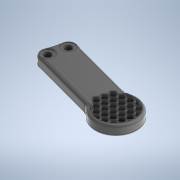
# Autodesk Inventor part: RearBumper
Saved by Autodesk Inventor 2020 (Build 240168000, 168)
## iProperties
Part Number: RearBumper
Material: PC/ABS プラスチック
Document SubType Name: Modeling
Designer: Masato Kubotera
Density: 0.357273 g/cm^3
Appearance: 滑らか - 黒
Description: TPU
Author: Masato Kubotera
Autodesk Inventor part; units mm, degrees
ref_plane "YZ Plane" through (0, 0, 0) normal (1, 0, 0) x (0, 1, 0)
ref_plane "XZ Plane" through (0, 0, 0) normal (0, 1, 0) x (-1, 0, 0)
ref_plane "XY Plane" through (0, 0, 0) normal (0, 0, 1) x (1, 0, 0)
derived "Trunk_basis.ipt"
sketch "スケッチ1" plane through (0, 0, 0) normal (0, 1, 0) x (-1, 0, 0)
  line L0 (0, 22) -> (0, -142.9) construction
  circle A0 centre (5, 0) radius 10.5 construction
  line L1 (-7, 16) -> (36, 16) construction
  line L2 (36, 16) -> (36, -16) construction
  line L3 (36, -16) -> (-7, -16) construction
  line L4 (-7, -16) -> (-7, 16) construction
  line L5 (-7, 16) -> (36, -16) construction
  line L6 (36, 16) -> (-7, -16) construction
  line L7 (33, 13.5) -> (6, 13.5) construction
  line L8 (6, 13.5) -> (6, -13.5) construction
  line L9 (6, -13.5) -> (33, -13.5) construction
  line L10 (33, -13.5) -> (33, 13.5) construction
  line L11 (33, 13.5) -> (6, -13.5) construction
  line L12 (6, 13.5) -> (33, -13.5) construction
  line L13 (-7, 0) -> (36, 0) construction
  arc A1 (5, 16) -> (-7, 10.583) centre (5, 0) ccw construction
  line L14 (43.75, -16.25) -> (5, -16.25)
  line L15 (5, 16.25) -> (43.75, 16.25)
  line L16 (44.75, 15.25) -> (44.75, -15.25)
  arc A2 (5, 16.25) -> (-6.7376, 11.2379) centre (5, 0) ccw
  arc A3 (-6.7376, 11.2379) -> (-7.25, 9.9174) centre (-6.2711, 10.2972) ccw
  circle A4 centre (6, 13.5) radius 1.35
  line L17 (19.5, 13.5) -> (19.5, -13.5) construction
  circle A5 centre (33, 13.5) radius 1.35
  line L18 (-15, 22) -> (-20, 17)
  line L19 (-20, 17) -> (-20, -19)
  line L20 (-20, -19) -> (-28.5, -27.5)
  line L21 (-28.5, -27.5) -> (-28.5, -103)
  line L22 (57.5, -22.5) -> (57.5, 17)
  line L23 (57.5, 17) -> (52.5, 22)
  line L24 (52.5, 22) -> (-15, 22)
  line L25 (-35.5597, -116.5529) -> (-28.5, -142.9)
  line L26 (-16, -139) -> (-16, -94) construction
  line L27 (-7.5, -140.4849) -> (-7.5, -142.9)
  line L28 (-7.5, -142.9) -> (7.5, -142.9)
  line L29 (7.5, -140.4849) -> (7.5, -142.9)
  arc A6 (-7.5, -140.4849) -> (-8.9849, -139) centre (-8.2425, -139.7425) ccw
  line L30 (-17.5, -138.9955) -> (-17.5, -133) construction
  line L31 (-19, -133) -> (-16, -133) construction
  line L32 (-19, -133) -> (-19, -139) construction
  line L33 (-16, -133) -> (-16, -139) construction
  line L34 (-15, 22) -> (-10, 22) construction
  line L35 (-10, 22) -> (-10, -22) construction
  line L36 (-10, -22) -> (-15, -22) construction
  line L37 (-15, -22) -> (-15, 22) construction
  line L38 (-15, 22) -> (-10, -22) construction
  line L39 (-10, 22) -> (-15, -22) construction
  line L40 (-12.5, 22) -> (-12.5, -22) construction
  line L41 (-10, 0) -> (-15, 0) construction
  circle A7 centre (-12.5, 17.75) radius 1.6
  line L42 (-15, 10) -> (-12.5, 10) construction
  line L43 (-12.5, 10) -> (-12.5, -10) construction
  line L44 (-12.5, -10) -> (-15, -10) construction
  line L45 (-15, -10) -> (-15, 10) construction
  line L46 (-15, 10) -> (-12.5, -10) construction
  line L47 (-12.5, 10) -> (-15, -10) construction
  line L48 (-12.25, 10.25) -> (-15.25, 10.25)
  line L49 (-15.25, 8.15) -> (-15.25, -8.15)
  line L50 (-15.25, -10.25) -> (-12.25, -10.25)
  line L51 (-12.25, -8.15) -> (-12.25, 8.15)
  line L52 (-12.25, 10.25) -> (-15.25, -10.25) construction
  line L53 (-15.25, 10.25) -> (-12.25, -10.25) construction
  arc A8 (-15.25, 10.25) -> (-15.25, 8.15) centre (-15.25, 9.2) ccw
  line L54 (-13.75, 10) -> (-13.75, -10) construction
  arc A9 (-12.25, 8.15) -> (-12.25, 10.25) centre (-12.25, 9.2) ccw
  circle A10 centre (-12.5, -17.75) radius 1.6
  arc A11 (-15.25, -8.15) -> (-15.25, -10.25) centre (-15.25, -9.2) ccw
  arc A12 (-12.25, -10.25) -> (-12.25, -8.15) centre (-12.25, -9.2) ccw
  line L55 (36, 14.4) -> (44.5, 14.4) construction
  line L56 (44.5, 14.4) -> (44.5, -14.4) construction
  line L57 (36, -14.4) -> (44.5, -14.4) construction
  line L58 (49.95, 7.95) -> (49.95, -7.95)
  line L59 (52.5, 0) -> (47.5, 0) construction
  line L60 (47.5, 22) -> (52.5, 22) construction
  line L61 (52.55, -7.95) -> (52.55, 7.95)
  line L62 (51.25, 10) -> (51.25, -10) construction
  line L63 (52.5, 10) -> (50, -10) construction
  line L64 (52.5, -10) -> (50, -10) construction
  line L65 (52.5, 10) -> (52.5, -10) construction
  line L66 (50, 10) -> (52.5, -10) construction
  line L67 (49.95, -10.05) -> (52.55, -10.05)
  line L68 (49.95, 10.05) -> (52.55, -10.05) construction
  line L69 (52.55, 10.05) -> (49.95, -10.05) construction
  line L70 (52.5, -22) -> (47.5, -22) construction
  line L71 (47.5, 22) -> (52.5, -22) construction
  line L72 (52.5, 22) -> (52.5, -22) construction
  line L73 (52.5, 22) -> (47.5, -22) construction
  line L74 (50, 22) -> (50, -22) construction
  line L75 (47.5, -22) -> (47.5, 22) construction
  circle A13 centre (50, -17.75) radius 1.6
  arc A14 (52.55, -10.05) -> (52.55, -7.95) centre (52.55, -9) ccw
  line L76 (50, -10) -> (50, 10) construction
  arc A15 (49.95, -7.95) -> (49.95, -10.05) centre (49.95, -9) ccw
  arc A16 (49.95, 10.05) -> (49.95, 7.95) centre (49.95, 9) ccw
  arc A17 (52.55, 7.95) -> (52.55, 10.05) centre (52.55, 9) ccw
  line L77 (50, 10) -> (52.5, 10) construction
  line L78 (52.55, 10.05) -> (49.95, 10.05)
  circle A18 centre (50, 17.75) radius 1.6
  circle A19 centre (5, 0) radius 16 construction
  arc A20 (-6.7376, -11.2379) -> (5, -16.25) centre (5, 0) ccw
  arc A21 (-7.25, -9.9174) -> (-6.7376, -11.2379) centre (-6.2711, -10.2972) ccw
  line L79 (-7.25, -9.9174) -> (-7.25, 9.9174)
  line L80 (17.5, -138.9955) -> (17.5, -133) construction
  line L81 (19, -133) -> (19, -139) construction
  line L82 (16, -133) -> (16, -139) construction
  line L83 (19, -133) -> (16, -133) construction
  circle A22 centre (6, -13.5) radius 1.35
  circle A23 centre (33, -13.5) radius 1.35
  line L84 (-25.5, -142.9) -> (-7.5, -142.9) construction
  line L85 (25.5, -142.9) -> (7.5, -142.9) construction
  line L86 (-23.5, -22.5) -> (57.5, -22.5) construction
  line L87 (57.5, -22.5) -> (57.5, -103)
  circle A24 centre (-13.5, -55) radius 1.75
  line L88 (-16.5, -59) -> (45.5, -59)
  line L89 (47.5, -61) -> (47.5, -82.5)
  line L90 (45.5, -84.5) -> (-16.5, -84.5)
  line L91 (-18.5, -82.5) -> (-18.5, -61)
  line L92 (-18.5, -59) -> (47.5, -84.5) construction
  line L93 (47.5, -59) -> (-18.5, -84.5) construction
  line L94 (-16.5, -27.5) -> (45.5, -27.5)
  line L95 (47.5, -29.5) -> (47.5, -49)
  line L96 (45.5, -51) -> (-16.5, -51)
  line L97 (-18.5, -49) -> (-18.5, -29.5)
  line L98 (-18.5, -27.5) -> (47.5, -51) construction
  line L99 (47.5, -27.5) -> (-18.5, -51) construction
  line L100 (-23.5, -108) -> (-28.5, -103)
  circle A25 centre (-20.5415, -102) radius 1.6
  line L101 (-25.7227, -96) -> (25.7227, -96)
  line L102 (25.7227, -96) -> (34.9603, -112)
  line L103 (35.5597, -116.5529) -> (28.5, -142.9)
  line L104 (-25.7227, -96) -> (-34.9603, -112)
  line L105 (57.5, -103) -> (52.5, -108)
  arc A26 (-16.5, -27.5) -> (-18.5, -29.5) centre (-16.5, -29.5) ccw
  arc A27 (-18.5, -49) -> (-16.5, -51) centre (-16.5, -49) ccw
  arc A28 (45.5, -51) -> (47.5, -49) centre (45.5, -49) ccw
  arc A29 (47.5, -29.5) -> (45.5, -27.5) centre (45.5, -29.5) ccw
  arc A30 (-16.5, -59) -> (-18.5, -61) centre (-16.5, -61) ccw
  arc A31 (-18.5, -82.5) -> (-16.5, -84.5) centre (-16.5, -82.5) ccw
  arc A32 (45.5, -84.5) -> (47.5, -82.5) centre (45.5, -82.5) ccw
  arc A33 (47.5, -61) -> (45.5, -59) centre (45.5, -61) ccw
  line L106 (-23.5, -108) -> (52.5, -108)
  line L107 (-25.5, -139) -> (-25.5, -142.9)
  line L108 (-25.5, -142.9) -> (-28.5, -142.9)
  line L109 (-17.9813, -99.3843) -> (-16.9961, -101.0907)
  line L110 (-16.9961, -102.9093) -> (-17.9813, -104.6157)
  line L111 (-19.5563, -105.525) -> (-21.5266, -105.525)
  line L112 (-23.1016, -104.6157) -> (-24.0868, -102.9093)
  line L113 (-24.0868, -101.0907) -> (-23.1016, -99.3843)
  line L114 (-21.5266, -98.475) -> (-19.5563, -98.475)
  line L115 (-16, -94) -> (16, -94) construction
  arc A34 (-24.0868, -101.0907) -> (-24.0868, -102.9093) centre (-23.5618, -102) ccw
  arc A35 (-23.1016, -104.6157) -> (-21.5266, -105.525) centre (-22.0516, -104.6157) ccw
  arc A36 (-19.5563, -105.525) -> (-17.9813, -104.6157) centre (-19.0313, -104.6157) ccw
  arc A37 (-16.9961, -102.9093) -> (-16.9961, -101.0907) centre (-17.5211, -102) ccw
  arc A38 (-17.9813, -99.3843) -> (-19.5563, -98.475) centre (-19.0313, -99.3843) ccw
  arc A39 (-21.5266, -98.475) -> (-23.1016, -99.3843) centre (-22.0516, -99.3843) ccw
  line L116 (16, -139) -> (16, -94) construction
  line L117 (16, -94) -> (-16, -94) construction
  line L118 (-25.5, -139) -> (-8.9849, -139)
  line L119 (25.5, -142.9) -> (28.5, -142.9)
  arc A40 (8.9849, -139) -> (7.5, -140.4849) centre (8.2425, -139.7425) ccw
  circle A41 centre (29.7641, -115) radius 1.25
  line L120 (33.4891, -124.2803) -> (21.898, -121.1745) construction
  line L121 (29.7641, -115) -> (25.623, -130.4548) construction
  circle A42 centre (29.7641, -115) radius 6 construction
  circle A43 centre (-20.5415, -102) radius 6 construction
  line L122 (1.9319, -109.4824) -> (7.5588, -130.4824)
  line L123 (5.6269, -133) -> (-5.6269, -133)
  line L124 (5.3151, -110.5176) -> (10.942, -131.5176)
  line L125 (12.8739, -133) -> (17.1947, -133)
  line L126 (19.1266, -131.5176) -> (24.7535, -110.5176)
  line L127 (22.8217, -108) -> (7.2469, -108)
  circle A44 centre (25.623, -130.4548) radius 1.25
  circle A45 centre (25.623, -130.4548) radius 6 construction
  line L128 (-1.9319, -109.4824) -> (-7.5588, -130.4824)
  arc A46 (1.9319, -109.4824) -> (-1.9319, -109.4824) centre (0, -110) ccw
  arc A47 (-7.5588, -130.4824) -> (-5.6269, -133) centre (-5.6269, -131) ccw
  arc A48 (5.6269, -133) -> (7.5588, -130.4824) centre (5.6269, -131) ccw
  arc A49 (7.2469, -108) -> (5.3151, -110.5176) centre (7.2469, -110) ccw
  arc A50 (24.7535, -110.5176) -> (22.8217, -108) centre (22.8217, -110) ccw
  arc A51 (17.1947, -133) -> (19.1266, -131.5176) centre (17.1947, -131) ccw
  arc A52 (10.942, -131.5176) -> (12.8739, -133) centre (12.8739, -131) ccw
  arc A53 (-5.3151, -110.5176) -> (-7.2469, -108) centre (-7.2469, -110) ccw
  line L129 (-22.8217, -108) -> (-7.2469, -108)
  line L130 (-5.3151, -110.5176) -> (-10.942, -131.5176)
  arc A54 (-22.8217, -108) -> (-24.7535, -110.5176) centre (-22.8217, -110) ccw
  line L131 (-19.1266, -131.5176) -> (-24.7535, -110.5176)
  arc A55 (-19.1266, -131.5176) -> (-17.1947, -133) centre (-17.1947, -131) ccw
  line L132 (-12.8739, -133) -> (-17.1947, -133)
  arc A56 (-12.8739, -133) -> (-10.942, -131.5176) centre (-12.8739, -131) ccw
  circle A57 centre (-29.7641, -115) radius 1.25
  circle A58 centre (-25.623, -130.4548) radius 1.25
  arc A59 (35.5597, -116.5529) -> (34.9603, -112) centre (29.7641, -115) ccw
  arc A60 (-34.9603, -112) -> (-35.5597, -116.5529) centre (-29.7641, -115) ccw
  arc A61 (-24.0151, -139) -> (-25.5, -140.4849) centre (-24.7575, -139.7425) ccw
  line L133 (25.5, -139) -> (25.5, -142.9)
  arc A62 (25.5, -140.4849) -> (24.0151, -139) centre (24.7575, -139.7425) ccw
  line L134 (25.5, -139) -> (8.9849, -139)
  line L135 (21.5266, -98.475) -> (19.5563, -98.475)
  line L136 (16.9961, -102.9093) -> (17.9813, -104.6157)
  arc A63 (21.5266, -105.525) -> (23.1016, -104.6157) centre (22.0516, -104.6157) ccw
  circle A64 centre (20.5415, -102) radius 1.6
  line L137 (24.0868, -101.0907) -> (23.1016, -99.3843)
  arc A65 (24.0868, -102.9093) -> (24.0868, -101.0907) centre (23.5618, -102) ccw
  line L138 (23.1016, -104.6157) -> (24.0868, -102.9093)
  arc A66 (23.1016, -99.3843) -> (21.5266, -98.475) centre (22.0516, -99.3843) ccw
  line L139 (19.5563, -105.525) -> (21.5266, -105.525)
  arc A67 (19.5563, -98.475) -> (17.9813, -99.3843) centre (19.0313, -99.3843) ccw
  arc A68 (17.9813, -104.6157) -> (19.5563, -105.525) centre (19.0313, -104.6157) ccw
  line L140 (17.9813, -99.3843) -> (16.9961, -101.0907)
  arc A69 (16.9961, -101.0907) -> (16.9961, -102.9093) centre (17.5211, -102) ccw
  line L141 (16, -139) -> (16, -94) construction
  circle A70 centre (20.5415, -102) radius 6 construction
  arc A71 (29.5045, -117.5445) -> (31.2612, -117.0738) centre (30.247, -116.802) ccw construction
  line L142 (31.8379, -116.4971) -> (31.2612, -117.0738) construction
  line L143 (29.5045, -117.5445) -> (28.7167, -117.3334) construction
  arc A72 (27.4307, -116.0474) -> (28.7167, -117.3334) centre (28.4449, -116.3192) ccw construction
  line L144 (27.4307, -116.0474) -> (27.2196, -115.2596) construction
  line L145 (27.6903, -113.5029) -> (28.267, -112.9262) construction
  arc A73 (30.0237, -112.4555) -> (28.267, -112.9262) centre (29.2813, -113.198) ccw construction
  arc A74 (27.6903, -113.5029) -> (27.2196, -115.2596) centre (27.9621, -114.5171) ccw construction
  line L146 (30.0237, -112.4555) -> (30.8116, -112.6666) construction
  arc A75 (31.8379, -116.4971) -> (32.3086, -114.7404) centre (31.5662, -115.4829) ccw construction
  arc A76 (32.0975, -113.9526) -> (30.8116, -112.6666) centre (31.0833, -113.6808) ccw construction
  line L147 (32.0975, -113.9526) -> (32.3086, -114.7404) construction
  line L148 (-20.5415, -102) -> (20.5415, -102) construction
  circle A77 centre (0, -102) radius 1.6
  line L149 (0.4078, -104.525) -> (-0.4078, -104.525)
  arc A78 (-0.4078, -99.475) -> (-1.9828, -100.3843) centre (-0.9328, -100.3843) ccw
  arc A79 (0.4078, -104.525) -> (1.9828, -103.6157) centre (0.9328, -103.6157) ccw
  line L150 (2.3906, -102.9093) -> (1.9828, -103.6157)
  line L151 (-0.4078, -99.475) -> (0.4078, -99.475)
  arc A80 (1.9828, -100.3843) -> (0.4078, -99.475) centre (0.9328, -100.3843) ccw
  line L152 (1.9828, -100.3843) -> (2.3906, -101.0907)
  arc A81 (2.3906, -102.9093) -> (2.3906, -101.0907) centre (1.8656, -102) ccw
  line L153 (-2.3906, -101.0907) -> (-1.9828, -100.3843)
  arc A82 (-2.3906, -101.0907) -> (-2.3906, -102.9093) centre (-1.8656, -102) ccw
  line L154 (-1.9828, -103.6157) -> (-2.3906, -102.9093)
  arc A83 (-1.9828, -103.6157) -> (-0.4078, -104.525) centre (-0.9328, -103.6157) ccw
  circle A84 centre (0, -102) radius 1.25
  arc A85 (44.75, 15.25) -> (43.75, 16.25) centre (43.75, 15.25) ccw
  arc A86 (43.75, -16.25) -> (44.75, -15.25) centre (43.75, -15.25) ccw
  point P0 (0, 0)
  point P1 (14.5, 0)
  point P2 (19.5, 0)
  point P3 (44.75, 16.25)
  point P4 (-7.25, 10.6771)
  point P5 (19.5, 0)
  point P6 (-12.5, 0)
  point P7 (-13.75, 0)
  point P8 (44.75, 14.4)
  point P9 (44.75, -14.4)
  point P10 (51.25, 0)
  point P11 (50, 0)
  point P12 (44.75, -16.25)
  point P13 (14.5, -71.75)
  point P14 (14.5, -39.25)
  point P15 (-18.5063, -98.475)
  point P16 (-16.4711, -102)
  point P17 (-18.5063, -105.525)
  point P18 (-22.5766, -105.525)
  point P19 (-22.5766, -98.475)
  point P20 (-24.6118, -102)
  point P21 (-22.5766, -105.525)
  point P22 (-18.5063, -105.525)
  point P23 (-16.4711, -102)
  point P24 (-18.5063, -98.475)
  point P25 (-22.5766, -98.475)
  point P26 (27.6936, -122.7274)
  point P27 (0, -102.2726)
  point P28 (0, -133)
  point P29 (-7.5, -139)
  point P30 (-22.5766, -98.475)
  point P31 (18.5063, -98.475)
  point P32 (18.5063, -98.475)
  point P33 (22.5766, -105.525)
  point P34 (22.5766, -105.525)
  point P35 (24.6118, -102)
  point P36 (22.5766, -98.475)
  point P37 (22.5766, -98.475)
  point P38 (22.5766, -98.475)
  point P39 (18.5063, -105.525)
  point P40 (16.4711, -102)
  point P41 (16.4711, -102)
  point P42 (18.5063, -105.525)
  point P43 (29.7641, -115)
  point P44 (29.7641, -115)
  point P45 (30.5187, -117.8163)
  point P46 (30.5187, -117.8163)
  point P47 (27.7025, -117.0617)
  point P48 (27.7025, -117.0617)
  point P49 (31.8258, -112.9383)
  point P50 (26.9479, -114.2454)
  point P51 (29.0095, -112.1837)
  point P52 (29.0095, -112.1837)
  point P53 (31.8258, -112.9383)
  point P54 (29.0095, -112.1837)
  point P55 (32.5804, -115.7546)
  point P56 (-1.4578, -99.475)
  point P57 (-1.4578, -99.475)
  point P58 (-1.4578, -99.475)
  point P59 (1.4578, -104.525)
  point P60 (1.4578, -99.475)
  point P61 (1.4578, -99.475)
  point P62 (2.9156, -102)
  point P63 (-2.9156, -102)
  point P64 (-1.4578, -104.525)
  point P65 (-1.4578, -104.525)
sketch "スケッチ2" plane through (0, 0, 0) normal (0, 1, 0) x (-1, 0, 0)
  circle A0 centre (29.7641, -115) radius 1.25 projected
  circle A1 centre (25.623, -130.4548) radius 1.25 projected
  circle A2 centre (29.7641, -115) radius 3.25
  arc A3 (31.5759, -108.2385) -> (23.0026, -113.1883) centre (29.7641, -115) ccw
  line L0 (31.5759, -108.2385) -> (93.8823, -124.9335)
  line L1 (33.4891, -124.2803) -> (21.898, -121.1745) construction
  circle A4 centre (25.623, -130.4548) radius 3.25
  arc A5 (18.8615, -128.6431) -> (23.8113, -137.2163) centre (25.623, -130.4548) ccw
  line L2 (23.8113, -137.2163) -> (86.1177, -153.9113)
  line L3 (0, 22) -> (0, -142.9) construction
  line L4 (23.0026, -113.1883) -> (18.8615, -128.6431)
  circle A6 centre (29.7641, -115) radius 6
  circle A7 centre (25.623, -130.4548) radius 6
  arc A8 (86.1177, -153.9113) -> (93.8823, -124.9335) centre (102.778, -142.8462) ccw
  arc A9 (86.1177, -153.9113) -> (93.8823, -124.9335) centre (90, -139.4224) ccw
  arc A10 (88.5278, -153.0041) -> (95.516, -126.9241) centre (102.778, -142.8462) ccw
  line L5 (91.3245, -139.7773) -> (88.875, -142.2268)
  line L6 (88.875, -142.2268) -> (85.529, -141.3302)
  line L7 (85.529, -141.3302) -> (84.6324, -137.9841)
  line L8 (84.6324, -137.9841) -> (87.0819, -135.5346)
  line L9 (87.0819, -135.5346) -> (90.4279, -136.4312)
  line L10 (90.4279, -136.4312) -> (91.3245, -139.7773)
  line L11 (85.0807, -139.6571) -> (90.8762, -138.1042) construction
  line L12 (85.8571, -136.7594) -> (90.0998, -141.002) construction
  line L13 (84.6324, -137.9841) -> (91.3245, -139.7773) construction
  line L14 (91.0075, -136.2759) -> (93.457, -133.8264)
  line L15 (91.9041, -139.622) -> (91.0075, -136.2759)
  line L16 (95.2501, -140.5186) -> (91.9041, -139.622)
  line L17 (97.6996, -138.0691) -> (95.2501, -140.5186)
  line L18 (96.8031, -134.723) -> (97.6996, -138.0691)
  line L19 (93.457, -133.8264) -> (96.8031, -134.723)
  line L20 (89.2993, -142.651) -> (91.7488, -140.2015)
  line L21 (90.1959, -145.9971) -> (89.2993, -142.651)
  line L22 (93.5419, -146.8937) -> (90.1959, -145.9971)
  line L23 (95.9914, -144.4442) -> (93.5419, -146.8937)
  line L24 (95.0948, -141.0981) -> (95.9914, -144.4442)
  line L25 (91.7488, -140.2015) -> (95.0948, -141.0981)
  line L26 (98.1239, -138.4933) -> (101.47, -139.3899)
  line L27 (95.6744, -140.9428) -> (98.1239, -138.4933)
  line L28 (96.571, -144.2889) -> (95.6744, -140.9428)
  line L29 (99.917, -145.1855) -> (96.571, -144.2889)
  line L30 (102.3665, -142.736) -> (99.917, -145.1855)
  line L31 (101.47, -139.3899) -> (102.3665, -142.736)
  line L32 (102.7908, -143.1602) -> (106.1369, -144.0568)
  line L33 (100.3413, -145.6097) -> (102.7908, -143.1602)
  line L34 (101.2379, -148.9558) -> (100.3413, -145.6097)
  line L35 (104.5839, -149.8524) -> (101.2379, -148.9558)
  line L36 (107.0334, -147.4029) -> (104.5839, -149.8524)
  line L37 (106.1369, -144.0568) -> (107.0334, -147.4029)
  line L38 (106.2922, -143.4773) -> (102.9461, -142.5807)
  line L39 (108.7416, -141.0278) -> (106.2922, -143.4773)
  line L40 (107.8451, -137.6817) -> (108.7416, -141.0278)
  line L41 (104.499, -136.7851) -> (107.8451, -137.6817)
  line L42 (102.0495, -139.2346) -> (104.499, -136.7851)
  line L43 (102.9461, -142.5807) -> (102.0495, -139.2346)
  line L44 (109.1659, -141.452) -> (112.512, -142.3486)
  line L45 (106.7164, -143.9015) -> (109.1659, -141.452)
  line L46 (107.613, -147.2476) -> (106.7164, -143.9015)
  line L47 (110.9591, -148.1442) -> (107.613, -147.2476)
  line L48 (113.4085, -145.6947) -> (110.9591, -148.1442)
  line L49 (112.512, -142.3486) -> (113.4085, -145.6947)
  line L50 (113.8328, -146.1189) -> (117.1789, -147.0155)
  line L51 (111.3833, -148.5684) -> (113.8328, -146.1189)
  line L52 (112.2799, -151.9145) -> (111.3833, -148.5684)
  line L53 (115.626, -152.8111) -> (112.2799, -151.9145)
  line L54 (118.0755, -150.3616) -> (115.626, -152.8111)
  line L55 (117.1789, -147.0155) -> (118.0755, -150.3616)
  line L56 (117.3342, -146.4359) -> (113.9881, -145.5394)
  line L57 (119.7837, -143.9865) -> (117.3342, -146.4359)
  line L58 (118.8871, -140.6404) -> (119.7837, -143.9865)
  line L59 (115.541, -139.7438) -> (118.8871, -140.6404)
  line L60 (113.0915, -142.1933) -> (115.541, -139.7438)
  line L61 (113.9881, -145.5394) -> (113.0915, -142.1933)
  line L62 (120.2079, -144.4107) -> (123.554, -145.3073)
  line L63 (117.7584, -146.8602) -> (120.2079, -144.4107)
  line L64 (118.655, -150.2063) -> (117.7584, -146.8602)
  line L65 (122.0011, -151.1029) -> (118.655, -150.2063)
  line L66 (124.4506, -148.6534) -> (122.0011, -151.1029)
  line L67 (123.554, -145.3073) -> (124.4506, -148.6534)
  line L68 (124.8748, -149.0776) -> (128.2209, -149.9742)
  line L69 (122.4253, -151.5271) -> (124.8748, -149.0776)
  line L70 (123.3219, -154.8732) -> (122.4253, -151.5271)
  line L71 (126.668, -155.7698) -> (123.3219, -154.8732)
  line L72 (129.1175, -153.3203) -> (126.668, -155.7698)
  line L73 (128.2209, -149.9742) -> (129.1175, -153.3203)
  line L74 (128.3762, -149.3946) -> (125.0301, -148.4981)
  line L75 (130.8257, -146.9452) -> (128.3762, -149.3946)
  line L76 (129.9291, -143.5991) -> (130.8257, -146.9452)
  line L77 (126.583, -142.7025) -> (129.9291, -143.5991)
  line L78 (124.1335, -145.152) -> (126.583, -142.7025)
  line L79 (125.0301, -148.4981) -> (124.1335, -145.152)
  line L80 (90.5832, -135.8516) -> (87.2372, -134.9551)
  line L81 (87.2372, -134.9551) -> (86.3406, -131.609)
  line L82 (86.3406, -131.609) -> (88.7901, -129.1595)
  line L83 (88.7901, -129.1595) -> (92.1361, -130.0561)
  line L84 (92.1361, -130.0561) -> (93.0327, -133.4022)
  line L85 (93.0327, -133.4022) -> (90.5832, -135.8516)
  line L86 (92.7157, -129.9008) -> (95.1652, -127.4513)
  line L87 (93.6123, -133.2469) -> (92.7157, -129.9008)
  line L88 (96.9583, -134.1434) -> (93.6123, -133.2469)
  line L89 (99.4078, -131.694) -> (96.9583, -134.1434)
  line L90 (98.5113, -128.3479) -> (99.4078, -131.694)
  line L91 (95.1652, -127.4513) -> (98.5113, -128.3479)
  line L92 (97.3826, -134.5677) -> (99.8321, -132.1182)
  line L93 (99.8321, -132.1182) -> (103.1782, -133.0148)
  line L94 (98.2792, -137.9138) -> (97.3826, -134.5677)
  line L95 (101.6252, -138.8103) -> (98.2792, -137.9138)
  line L96 (104.0747, -136.3609) -> (101.6252, -138.8103)
  line L97 (103.1782, -133.0148) -> (104.0747, -136.3609)
  line L98 (104.6543, -136.2056) -> (103.7577, -132.8595)
  line L99 (103.7577, -132.8595) -> (106.2072, -130.41)
  line L100 (106.2072, -130.41) -> (109.5533, -131.3066)
  line L101 (109.5533, -131.3066) -> (110.4499, -134.6527)
  line L102 (110.4499, -134.6527) -> (108.0004, -137.1021)
  line L103 (108.0004, -137.1021) -> (104.6543, -136.2056)
  line L104 (108.4246, -137.5264) -> (110.8741, -135.0769)
  line L105 (110.8741, -135.0769) -> (114.2202, -135.9735)
  line L106 (114.2202, -135.9735) -> (115.1168, -139.3196)
  line L107 (115.1168, -139.3196) -> (112.6673, -141.769)
  line L108 (112.6673, -141.769) -> (109.3212, -140.8725)
  line L109 (109.3212, -140.8725) -> (108.4246, -137.5264)
  line L110 (115.6963, -139.1643) -> (114.7997, -135.8182)
  line L111 (114.7997, -135.8182) -> (117.2492, -133.3687)
  line L112 (117.2492, -133.3687) -> (120.5953, -134.2653)
  line L113 (120.5953, -134.2653) -> (121.4919, -137.6113)
  line L114 (121.4919, -137.6113) -> (119.0424, -140.0608)
  line L115 (119.0424, -140.0608) -> (115.6963, -139.1643)
  line L116 (120.3632, -143.8312) -> (119.4666, -140.4851)
  line L117 (119.4666, -140.4851) -> (121.9161, -138.0356)
  line L118 (121.9161, -138.0356) -> (125.2622, -138.9322)
  line L119 (125.2622, -138.9322) -> (126.1588, -142.2783)
  line L120 (126.1588, -142.2783) -> (123.7093, -144.7277)
  line L121 (123.7093, -144.7277) -> (120.3632, -143.8312)
  line L122 (130.0844, -143.0195) -> (126.7383, -142.123)
  line L123 (126.7383, -142.123) -> (125.8418, -138.7769)
  line L124 (125.8418, -138.7769) -> (128.2912, -136.3274)
  line L125 (128.2912, -136.3274) -> (131.6373, -137.224)
  line L126 (131.6373, -137.224) -> (132.5339, -140.57)
  line L127 (132.5339, -140.57) -> (130.0844, -143.0195)
  line L128 (92.2914, -129.4765) -> (88.9454, -128.58)
  line L129 (88.9454, -128.58) -> (88.0488, -125.2339)
  line L130 (88.0488, -125.2339) -> (90.4983, -122.7844)
  line L131 (90.4983, -122.7844) -> (93.8444, -123.681)
  line L132 (93.8444, -123.681) -> (94.7409, -127.027)
  line L133 (94.7409, -127.027) -> (92.2914, -129.4765)
  line L134 (94.4239, -123.5257) -> (96.8734, -121.0762)
  line L135 (95.3205, -126.8718) -> (94.4239, -123.5257)
  line L136 (98.6666, -127.7683) -> (95.3205, -126.8718)
  line L137 (101.116, -125.3188) -> (98.6666, -127.7683)
  line L138 (100.2195, -121.9728) -> (101.116, -125.3188)
  line L139 (96.8734, -121.0762) -> (100.2195, -121.9728)
  line L140 (99.0908, -128.1926) -> (101.5403, -125.7431)
  line L141 (101.5403, -125.7431) -> (104.8864, -126.6397)
  line L142 (99.9874, -131.5387) -> (99.0908, -128.1926)
  line L143 (103.3335, -132.4352) -> (99.9874, -131.5387)
  line L144 (105.7829, -129.9857) -> (103.3335, -132.4352)
  line L145 (104.8864, -126.6397) -> (105.7829, -129.9857)
  line L146 (106.3625, -129.8305) -> (105.4659, -126.4844)
  line L147 (105.4659, -126.4844) -> (107.9154, -124.0349)
  line L148 (107.9154, -124.0349) -> (111.2615, -124.9315)
  line L149 (111.2615, -124.9315) -> (112.1581, -128.2775)
  line L150 (112.1581, -128.2775) -> (109.7086, -130.727)
  line L151 (109.7086, -130.727) -> (106.3625, -129.8305)
  line L152 (110.1328, -131.1513) -> (112.5823, -128.7018)
  line L153 (112.5823, -128.7018) -> (115.9284, -129.5984)
  line L154 (115.9284, -129.5984) -> (116.825, -132.9444)
  line L155 (116.825, -132.9444) -> (114.3755, -135.3939)
  line L156 (114.3755, -135.3939) -> (111.0294, -134.4974)
  line L157 (111.0294, -134.4974) -> (110.1328, -131.1513)
  line L158 (117.4045, -132.7892) -> (116.5079, -129.4431)
  line L159 (116.5079, -129.4431) -> (118.9574, -126.9936)
  line L160 (118.9574, -126.9936) -> (122.3035, -127.8902)
  line L161 (122.3035, -127.8902) -> (123.2001, -131.2362)
  line L162 (123.2001, -131.2362) -> (120.7506, -133.6857)
  line L163 (120.7506, -133.6857) -> (117.4045, -132.7892)
  line L164 (122.0714, -137.4561) -> (121.1748, -134.11)
  line L165 (121.1748, -134.11) -> (123.6243, -131.6605)
  line L166 (123.6243, -131.6605) -> (126.9704, -132.5571)
  line L167 (126.9704, -132.5571) -> (127.867, -135.9031)
  line L168 (127.867, -135.9031) -> (125.4175, -138.3526)
  line L169 (125.4175, -138.3526) -> (122.0714, -137.4561)
  line L170 (131.7926, -136.6444) -> (128.4465, -135.7479)
  line L171 (128.4465, -135.7479) -> (127.55, -132.4018)
  line L172 (127.55, -132.4018) -> (129.9994, -129.9523)
  line L173 (129.9994, -129.9523) -> (133.3455, -130.8489)
  line L174 (133.3455, -130.8489) -> (134.2421, -134.1949)
  line L175 (134.2421, -134.1949) -> (131.7926, -136.6444)
  line L176 (89.6163, -146.1524) -> (87.1668, -148.6019)
  line L177 (88.7197, -142.8063) -> (89.6163, -146.1524)
  line L178 (85.3737, -141.9097) -> (88.7197, -142.8063)
  line L179 (82.9242, -144.3592) -> (85.3737, -141.9097)
  line L180 (83.8208, -147.7053) -> (82.9242, -144.3592)
  line L181 (87.1668, -148.6019) -> (83.8208, -147.7053)
  line L182 (87.5911, -149.0261) -> (90.0406, -146.5766)
  line L183 (90.0406, -146.5766) -> (93.3866, -147.4732)
  line L184 (93.3866, -147.4732) -> (94.2832, -150.8193)
  line L185 (94.2832, -150.8193) -> (91.8337, -153.2688)
  line L186 (91.8337, -153.2688) -> (88.4877, -152.3722)
  line L187 (88.4877, -152.3722) -> (87.5911, -149.0261)
  line L188 (98.6331, -151.9848) -> (101.0826, -149.5353)
  line L189 (99.5297, -155.3309) -> (98.6331, -151.9848)
  line L190 (100.6583, -149.1111) -> (98.2088, -151.5606)
  line L191 (98.2088, -151.5606) -> (94.8628, -150.664)
  line L192 (94.8628, -150.664) -> (93.9662, -147.3179)
  line L193 (93.9662, -147.3179) -> (96.4157, -144.8684)
  line L194 (96.4157, -144.8684) -> (99.7618, -145.765)
  line L195 (99.7618, -145.765) -> (100.6583, -149.1111)
  line L196 (101.0826, -149.5353) -> (104.4287, -150.4319)
  line L197 (104.4287, -150.4319) -> (105.3252, -153.778)
  line L198 (105.3252, -153.778) -> (102.8757, -156.2275)
  line L199 (102.8757, -156.2275) -> (99.5297, -155.3309)
  line L200 (109.2509, -154.5193) -> (105.9048, -153.6227)
  line L201 (105.9048, -153.6227) -> (105.0082, -150.2766)
  line L202 (105.0082, -150.2766) -> (107.4577, -147.8271)
  line L203 (107.4577, -147.8271) -> (110.8038, -148.7237)
  line L204 (110.8038, -148.7237) -> (111.7003, -152.0698)
  line L205 (111.7003, -152.0698) -> (109.2509, -154.5193)
  line L206 (112.1246, -152.494) -> (115.4707, -153.3906)
  line L207 (109.6751, -154.9435) -> (112.1246, -152.494)
  line L208 (110.5717, -158.2896) -> (109.6751, -154.9435)
  line L209 (113.9178, -159.1862) -> (110.5717, -158.2896)
  line L210 (116.3672, -156.7367) -> (113.9178, -159.1862)
  line L211 (115.4707, -153.3906) -> (116.3672, -156.7367)
  line L212 (122.7424, -155.0285) -> (120.2929, -157.478)
  line L213 (120.2929, -157.478) -> (116.9468, -156.5814)
  line L214 (116.0502, -153.2353) -> (118.4997, -150.7858)
  line L215 (116.9468, -156.5814) -> (116.0502, -153.2353)
  line L216 (118.4997, -150.7858) -> (121.8458, -151.6824)
  line L217 (121.8458, -151.6824) -> (122.7424, -155.0285)
  line L218 (120.7171, -157.9022) -> (123.1666, -155.4527)
  line L219 (123.1666, -155.4527) -> (126.5127, -156.3493)
  line L220 (126.5127, -156.3493) -> (127.4093, -159.6954)
  line L221 (127.4093, -159.6954) -> (124.9598, -162.1449)
  line L222 (124.9598, -162.1449) -> (121.6137, -161.2483)
  line L223 (121.6137, -161.2483) -> (120.7171, -157.9022)
  line L224 (87.9081, -152.5275) -> (85.4586, -154.977)
  line L225 (87.0115, -149.1814) -> (87.9081, -152.5275)
  line L226 (83.6655, -148.2848) -> (87.0115, -149.1814)
  line L227 (81.216, -150.7343) -> (83.6655, -148.2848)
  line L228 (82.1126, -154.0804) -> (81.216, -150.7343)
  line L229 (85.4586, -154.977) -> (82.1126, -154.0804)
  line L230 (85.8829, -155.4012) -> (88.3324, -152.9518)
  line L231 (88.3324, -152.9518) -> (91.6784, -153.8483)
  line L232 (91.6784, -153.8483) -> (92.575, -157.1944)
  line L233 (92.575, -157.1944) -> (90.1255, -159.6439)
  line L234 (90.1255, -159.6439) -> (86.7795, -158.7473)
  line L235 (86.7795, -158.7473) -> (85.8829, -155.4012)
  line L236 (96.9249, -158.3599) -> (99.3744, -155.9105)
  line L237 (97.8215, -161.706) -> (96.9249, -158.3599)
  line L238 (98.9501, -155.4862) -> (96.5006, -157.9357)
  line L239 (96.5006, -157.9357) -> (93.1546, -157.0391)
  line L240 (93.1546, -157.0391) -> (92.258, -153.693)
  line L241 (92.258, -153.693) -> (94.7075, -151.2435)
  line L242 (94.7075, -151.2435) -> (98.0535, -152.1401)
  line L243 (98.0535, -152.1401) -> (98.9501, -155.4862)
  line L244 (99.3744, -155.9105) -> (102.7205, -156.807)
  line L245 (102.7205, -156.807) -> (103.617, -160.1531)
  line L246 (103.617, -160.1531) -> (101.1675, -162.6026)
  line L247 (101.1675, -162.6026) -> (97.8215, -161.706)
  line L248 (107.5426, -160.8944) -> (104.1966, -159.9978)
  line L249 (104.1966, -159.9978) -> (103.3, -156.6517)
  line L250 (103.3, -156.6517) -> (105.7495, -154.2022)
  line L251 (105.7495, -154.2022) -> (109.0956, -155.0988)
  line L252 (109.0956, -155.0988) -> (109.9921, -158.4449)
  line L253 (109.9921, -158.4449) -> (107.5426, -160.8944)
  line L254 (110.4164, -158.8692) -> (113.7625, -159.7657)
  line L255 (107.9669, -161.3186) -> (110.4164, -158.8692)
  line L256 (108.8635, -164.6647) -> (107.9669, -161.3186)
  line L257 (112.2096, -165.5613) -> (108.8635, -164.6647)
  line L258 (114.659, -163.1118) -> (112.2096, -165.5613)
  line L259 (113.7625, -159.7657) -> (114.659, -163.1118)
  line L260 (121.0342, -161.4036) -> (118.5847, -163.8531)
  line L261 (118.5847, -163.8531) -> (115.2386, -162.9565)
  line L262 (114.342, -159.6104) -> (116.7915, -157.1609)
  line L263 (115.2386, -162.9565) -> (114.342, -159.6104)
  line L264 (116.7915, -157.1609) -> (120.1376, -158.0575)
  line L265 (120.1376, -158.0575) -> (121.0342, -161.4036)
  line L266 (119.0089, -164.2773) -> (121.4584, -161.8278)
  line L267 (121.4584, -161.8278) -> (124.8045, -162.7244)
  line L268 (124.8045, -162.7244) -> (125.7011, -166.0705)
  line L269 (125.7011, -166.0705) -> (123.2516, -168.52)
  line L270 (123.2516, -168.52) -> (119.9055, -167.6234)
  line L271 (119.9055, -167.6234) -> (119.0089, -164.2773)
  line L272 (86.1999, -158.9026) -> (83.7504, -161.3521)
  line L273 (85.3033, -155.5565) -> (86.1999, -158.9026)
  line L274 (81.9573, -154.66) -> (85.3033, -155.5565)
  line L275 (79.5078, -157.1094) -> (81.9573, -154.66)
  line L276 (80.4043, -160.4555) -> (79.5078, -157.1094)
  line L277 (83.7504, -161.3521) -> (80.4043, -160.4555)
  line L278 (84.1747, -161.7764) -> (86.6242, -159.3269)
  line L279 (86.6242, -159.3269) -> (89.9702, -160.2234)
  line L280 (89.9702, -160.2234) -> (90.8668, -163.5695)
  line L281 (90.8668, -163.5695) -> (88.4173, -166.019)
  line L282 (88.4173, -166.019) -> (85.0713, -165.1224)
  line L283 (85.0713, -165.1224) -> (84.1747, -161.7764)
  line L284 (95.2167, -164.7351) -> (97.6662, -162.2856)
  line L285 (96.1133, -168.0811) -> (95.2167, -164.7351)
  line L286 (97.2419, -161.8613) -> (94.7924, -164.3108)
  line L287 (94.7924, -164.3108) -> (91.4464, -163.4142)
  line L288 (91.4464, -163.4142) -> (90.5498, -160.0681)
  line L289 (90.5498, -160.0681) -> (92.9993, -157.6187)
  line L290 (92.9993, -157.6187) -> (96.3453, -158.5152)
  line L291 (96.3453, -158.5152) -> (97.2419, -161.8613)
  line L292 (97.6662, -162.2856) -> (101.0122, -163.1821)
  line L293 (101.0122, -163.1821) -> (101.9088, -166.5282)
  line L294 (101.9088, -166.5282) -> (99.4593, -168.9777)
  line L295 (99.4593, -168.9777) -> (96.1133, -168.0811)
  line L296 (105.8344, -167.2695) -> (102.4884, -166.3729)
  line L297 (102.4884, -166.3729) -> (101.5918, -163.0268)
  line L298 (101.5918, -163.0268) -> (104.0413, -160.5774)
  line L299 (104.0413, -160.5774) -> (107.3874, -161.4739)
  line L300 (107.3874, -161.4739) -> (108.2839, -164.82)
  line L301 (108.2839, -164.82) -> (105.8344, -167.2695)
  line L302 (108.7082, -165.2443) -> (112.0543, -166.1408)
  line L303 (106.2587, -167.6938) -> (108.7082, -165.2443)
  line L304 (107.1553, -171.0398) -> (106.2587, -167.6938)
  line L305 (110.5013, -171.9364) -> (107.1553, -171.0398)
  line L306 (112.9508, -169.4869) -> (110.5013, -171.9364)
  line L307 (112.0543, -166.1408) -> (112.9508, -169.4869)
  line L308 (119.3259, -167.7787) -> (116.8765, -170.2282)
  line L309 (116.8765, -170.2282) -> (113.5304, -169.3316)
  line L310 (112.6338, -165.9855) -> (115.0833, -163.5361)
  line L311 (113.5304, -169.3316) -> (112.6338, -165.9855)
  line L312 (115.0833, -163.5361) -> (118.4294, -164.4326)
  line L313 (118.4294, -164.4326) -> (119.3259, -167.7787)
  line L314 (117.3007, -170.6524) -> (119.7502, -168.203)
  line L315 (119.7502, -168.203) -> (123.0963, -169.0995)
  line L316 (123.0963, -169.0995) -> (123.9929, -172.4456)
  line L317 (123.9929, -172.4456) -> (121.5434, -174.8951)
  line L318 (121.5434, -174.8951) -> (118.1973, -173.9985)
  line L319 (118.1973, -173.9985) -> (117.3007, -170.6524)
  line L320 (93.9996, -123.1014) -> (90.6536, -122.2049)
  line L321 (90.6536, -122.2049) -> (89.757, -118.8588)
  line L322 (89.757, -118.8588) -> (92.2065, -116.4093)
  line L323 (92.2065, -116.4093) -> (95.5526, -117.3059)
  line L324 (95.5526, -117.3059) -> (96.4491, -120.6519)
  line L325 (96.4491, -120.6519) -> (93.9996, -123.1014)
  line L326 (96.1321, -117.1506) -> (98.5816, -114.7011)
  line L327 (97.0287, -120.4966) -> (96.1321, -117.1506)
  line L328 (100.3748, -121.3932) -> (97.0287, -120.4966)
  line L329 (102.8242, -118.9437) -> (100.3748, -121.3932)
  line L330 (101.9277, -115.5977) -> (102.8242, -118.9437)
  line L331 (98.5816, -114.7011) -> (101.9277, -115.5977)
  line L332 (100.799, -121.8175) -> (103.2485, -119.368)
  line L333 (103.2485, -119.368) -> (106.5946, -120.2646)
  line L334 (101.6956, -125.1635) -> (100.799, -121.8175)
  line L335 (105.0417, -126.0601) -> (101.6956, -125.1635)
  line L336 (107.4912, -123.6106) -> (105.0417, -126.0601)
  line L337 (106.5946, -120.2646) -> (107.4912, -123.6106)
  line L338 (108.0707, -123.4553) -> (107.1741, -120.1093)
  line L339 (107.1741, -120.1093) -> (109.6236, -117.6598)
  line L340 (109.6236, -117.6598) -> (112.9697, -118.5564)
  line L341 (112.9697, -118.5564) -> (113.8663, -121.9024)
  line L342 (113.8663, -121.9024) -> (111.4168, -124.3519)
  line L343 (111.4168, -124.3519) -> (108.0707, -123.4553)
  line L344 (111.841, -124.7762) -> (114.2905, -122.3267)
  line L345 (114.2905, -122.3267) -> (117.6366, -123.2233)
  line L346 (117.6366, -123.2233) -> (118.5332, -126.5693)
  line L347 (118.5332, -126.5693) -> (116.0837, -129.0188)
  line L348 (116.0837, -129.0188) -> (112.7376, -128.1222)
  line L349 (112.7376, -128.1222) -> (111.841, -124.7762)
  line L350 (119.1127, -126.414) -> (118.2161, -123.068)
  line L351 (118.2161, -123.068) -> (120.6656, -120.6185)
  line L352 (120.6656, -120.6185) -> (124.0117, -121.5151)
  line L353 (124.0117, -121.5151) -> (124.9083, -124.8611)
  line L354 (124.9083, -124.8611) -> (122.4588, -127.3106)
  line L355 (122.4588, -127.3106) -> (119.1127, -126.414)
  line L356 (123.7796, -131.0809) -> (122.8831, -127.7349)
  line L357 (122.8831, -127.7349) -> (125.3325, -125.2854)
  line L358 (125.3325, -125.2854) -> (128.6786, -126.182)
  line L359 (128.6786, -126.182) -> (129.5752, -129.528)
  line L360 (129.5752, -129.528) -> (127.1257, -131.9775)
  line L361 (127.1257, -131.9775) -> (123.7796, -131.0809)
  line L362 (133.5008, -130.2693) -> (130.1547, -129.3727)
  line L363 (130.1547, -129.3727) -> (129.2582, -126.0267)
  line L364 (129.2582, -126.0267) -> (131.7077, -123.5772)
  line L365 (131.7077, -123.5772) -> (135.0537, -124.4738)
  line L366 (135.0537, -124.4738) -> (135.9503, -127.8198)
  line L367 (135.9503, -127.8198) -> (133.5008, -130.2693)
  point P0 (0, 0)
  point P1 (87.9785, -138.8807)
  point P2 (92.2322, -135.0512)
  point P3 (91.4558, -137.9489)
  point P4 (96.4749, -139.2938)
  point P5 (97.2513, -136.396)
  point P6 (90.524, -141.4263)
  point P7 (89.7476, -144.3241)
  point P8 (94.7667, -145.6689)
  point P9 (95.5431, -142.7711)
  point P10 (96.8991, -139.7181)
  point P11 (96.1227, -142.6158)
  point P12 (101.1418, -143.9607)
  point P13 (101.9182, -141.0629)
  point P14 (101.5661, -144.385)
  point P15 (100.7896, -147.2828)
  point P16 (105.8087, -148.6276)
  point P17 (106.5852, -145.7298)
  point P18 (107.5169, -142.2525)
  point P19 (108.2934, -139.3547)
  point P20 (103.2743, -138.0099)
  point P21 (102.4978, -140.9076)
  point P22 (107.9412, -142.6768)
  point P23 (107.1647, -145.5745)
  point P24 (112.1838, -146.9194)
  point P25 (112.9603, -144.0216)
  point P26 (112.6081, -147.3437)
  point P27 (111.8316, -150.2415)
  point P28 (116.8507, -151.5863)
  point P29 (117.6272, -148.6885)
  point P30 (118.5589, -145.2112)
  point P31 (119.3354, -142.3134)
  point P32 (114.3163, -140.9686)
  point P33 (113.5398, -143.8663)
  point P34 (118.9832, -145.6355)
  point P35 (118.2067, -148.5332)
  point P36 (123.2258, -149.8781)
  point P37 (124.0023, -146.9803)
  point P38 (123.6501, -150.3024)
  point P39 (122.8736, -153.2002)
  point P40 (127.8927, -154.545)
  point P41 (128.6692, -151.6472)
  point P42 (129.6009, -148.1699)
  point P43 (130.3774, -145.2721)
  point P44 (125.3583, -143.9273)
  point P45 (124.5818, -146.825)
  point P46 (86.7889, -133.282)
  point P47 (87.5653, -130.3843)
  point P48 (92.5844, -131.7291)
  point P49 (91.808, -134.6269)
  point P50 (93.9404, -128.6761)
  point P51 (93.164, -131.5738)
  point P52 (98.1831, -132.9187)
  point P53 (98.9595, -130.0209)
  point P54 (98.6074, -133.343)
  point P55 (97.8309, -136.2407)
  point P56 (102.85, -137.5856)
  point P57 (103.6265, -134.6878)
  point P58 (104.206, -134.5325)
  point P59 (104.9825, -131.6348)
  point P60 (110.0016, -132.9796)
  point P61 (109.2251, -135.8774)
  point P62 (109.6494, -136.3017)
  point P63 (114.6685, -137.6465)
  point P64 (113.892, -140.5443)
  point P65 (108.8729, -139.1994)
  point P66 (115.248, -137.4912)
  point P67 (116.0245, -134.5935)
  point P68 (121.0436, -135.9383)
  point P69 (120.2671, -138.8361)
  point P70 (119.9149, -142.1581)
  point P71 (120.6914, -139.2604)
  point P72 (125.7105, -140.6052)
  point P73 (124.934, -143.503)
  point P74 (126.29, -140.4499)
  point P75 (127.0665, -137.5522)
  point P76 (132.0856, -138.897)
  point P77 (131.3091, -141.7948)
  point P78 (88.4971, -126.9069)
  point P79 (89.2735, -124.0092)
  point P80 (94.2926, -125.354)
  point P81 (93.5162, -128.2518)
  point P82 (95.6487, -122.3009)
  point P83 (94.8722, -125.1987)
  point P84 (99.8913, -126.5436)
  point P85 (100.6678, -123.6458)
  point P86 (100.3156, -126.9678)
  point P87 (99.5391, -129.8656)
  point P88 (104.5582, -131.2105)
  point P89 (105.3347, -128.3127)
  point P90 (105.9142, -128.1574)
  point P91 (106.6907, -125.2596)
  point P92 (111.7098, -126.6045)
  point P93 (110.9333, -129.5023)
  point P94 (111.3576, -129.9265)
  point P95 (116.3767, -131.2714)
  point P96 (115.6002, -134.1692)
  point P97 (110.5811, -132.8243)
  point P98 (116.9562, -131.1161)
  point P99 (117.7327, -128.2183)
  point P100 (122.7518, -129.5632)
  point P101 (121.9753, -132.461)
  point P102 (121.6231, -135.783)
  point P103 (122.3996, -132.8852)
  point P104 (127.4187, -134.2301)
  point P105 (126.6422, -137.1279)
  point P106 (127.9982, -134.0748)
  point P107 (128.7747, -131.177)
  point P108 (133.7938, -132.5219)
  point P109 (133.0173, -135.4197)
  point P110 (88.3916, -147.3771)
  point P111 (89.168, -144.4793)
  point P112 (84.1489, -143.1345)
  point P113 (83.3725, -146.0323)
  point P114 (88.8158, -147.8014)
  point P115 (93.8349, -149.1462)
  point P116 (93.0585, -152.044)
  point P117 (88.0394, -150.6992)
  point P118 (99.8578, -150.7601)
  point P119 (99.0814, -153.6579)
  point P120 (99.4336, -150.3358)
  point P121 (94.4145, -148.991)
  point P122 (95.1909, -146.0932)
  point P123 (100.21, -147.438)
  point P124 (104.8769, -152.1049)
  point P125 (104.1005, -155.0027)
  point P126 (105.4565, -151.9497)
  point P127 (106.233, -149.0519)
  point P128 (111.2521, -150.3967)
  point P129 (110.4756, -153.2945)
  point P130 (110.8999, -153.7188)
  point P131 (110.1234, -156.6166)
  point P132 (115.1425, -157.9614)
  point P133 (115.919, -155.0636)
  point P134 (121.5176, -156.2532)
  point P135 (117.275, -152.0106)
  point P136 (116.4985, -154.9084)
  point P137 (122.2941, -153.3554)
  point P138 (121.9419, -156.6775)
  point P139 (126.961, -158.0223)
  point P140 (126.1845, -160.9201)
  point P141 (121.1654, -159.5753)
  point P142 (86.6834, -153.7522)
  point P143 (87.4598, -150.8545)
  point P144 (82.4407, -149.5096)
  point P145 (81.6643, -152.4074)
  point P146 (87.1076, -154.1765)
  point P147 (92.1267, -155.5214)
  point P148 (91.3503, -158.4191)
  point P149 (86.3312, -157.0743)
  point P150 (98.1496, -157.1352)
  point P151 (97.3732, -160.033)
  point P152 (97.7254, -156.7109)
  point P153 (92.7063, -155.3661)
  point P154 (93.4827, -152.4683)
  point P155 (98.5018, -153.8132)
  point P156 (103.1687, -158.4801)
  point P157 (102.3923, -161.3778)
  point P158 (103.7483, -158.3248)
  point P159 (104.5248, -155.427)
  point P160 (109.5438, -156.7719)
  point P161 (108.7674, -159.6696)
  point P162 (109.1917, -160.0939)
  point P163 (108.4152, -162.9917)
  point P164 (113.4343, -164.3365)
  point P165 (114.2108, -161.4388)
  point P166 (119.8094, -162.6283)
  point P167 (115.5668, -158.3857)
  point P168 (114.7903, -161.2835)
  point P169 (120.5859, -159.7306)
  point P170 (120.2337, -163.0526)
  point P171 (125.2528, -164.3975)
  point P172 (124.4763, -167.2952)
  point P173 (119.4572, -165.9504)
  point P174 (84.9752, -160.1273)
  point P175 (85.7516, -157.2296)
  point P176 (80.7325, -155.8847)
  point P177 (79.9561, -158.7825)
  point P178 (85.3994, -160.5516)
  point P179 (90.4185, -161.8965)
  point P180 (89.6421, -164.7942)
  point P181 (84.623, -163.4494)
  point P182 (96.4414, -163.5103)
  point P183 (95.665, -166.4081)
  point P184 (96.0172, -163.086)
  point P185 (90.9981, -161.7412)
  point P186 (91.7745, -158.8434)
  point P187 (96.7936, -160.1883)
  point P188 (101.4605, -164.8552)
  point P189 (100.6841, -167.7529)
  point P190 (102.0401, -164.6999)
  point P191 (102.8165, -161.8021)
  point P192 (107.8356, -163.147)
  point P193 (107.0592, -166.0447)
  point P194 (107.4835, -166.469)
  point P195 (106.707, -169.3668)
  point P196 (111.7261, -170.7116)
  point P197 (112.5025, -167.8139)
  point P198 (118.1012, -169.0034)
  point P199 (113.8586, -164.7608)
  dimension "d1" = 6.5
  dimension "d2" = 7
  dimension "d6" = 12
  dimension "d57" = 20
  dimension "d65" = 2.5
  dimension "d89" = 6.6
  dimension "d96" = 6.6
  dimension "d103" = 11.4315
  dimension "d108" = 0.6
  dimension "d109" = 0.6
  dimension "d110" = 0.6
  dimension "d113" = 6.6
  dimension "d120" = 6.6
  dimension "d125" = 0.6
  dimension "d126" = 0.6
  dimension "d127" = 90
  dimension "d128" = 6
  constraints: 732 end point, 8 centre point, 8 point on circle, 5 symmetric about line, 4 coincident, 4 midpoint, 4 tangent, 2 point on line, 1 collinear, 1 parallel, 972 other
  measures "d1" diameter of A2
  measures "d2" radius of A3
  measures "d6" diameter of A6
  measures "d57" radius of A8
  measures "d89" distance of L7.end L14.start
  measures "d96" distance of L7.end L20.start
  measures "d103" distance of L8.end L26.start
  measures "d108" distance between parallel lines of L10 L15
  measures "d109" distance between parallel lines of L20 L5
  measures "d110" distance between parallel lines of L24 L28
  measures "d113" distance of L5.end L80.start
  measures "d120" distance of L5.start L176.start
  measures "d125" distance between parallel lines of L178 L6
  measures "d126" distance between parallel lines of L9 L80
  measures "d127" horizontal distance of L3.end A9.centre
  measures "d128" distance between parallel lines of L272 L275
extrude "押し出し1" add sketch "スケッチ2" along normal blind 10 contours L0 L130 L129 L128 L133 L132 A9 L135 L136 L137 L140 L142 L143 L98 L41 L42 L43 L38 L32 L33 L34 L35 L188 L242 L241 L240 L232 L231 L230 L224 L225 L226 L227 L228 L2 A5 L4 A3 | L0 A9 L132 L133 L128 L129 L130 | A8 L132 A9 | A8 L135 A9 L132 | L228 L227 L226 L225 L224 A9 L2 | A8 L138 L137 A10 A9 L135 | A9 A10 L136 L135 | A9 L224 A8 | A8 L334 L335 A10 L137 L138 | L224 A9 L230 A8 | A8 L337 L336 A10 L335 L334 | L137 A10 L335 L336 L147 L146 L151 L150 L149 L153 L152 L157 L156 L155 L154 L112 L111 L110 L115 L114 L117 L116 L63 L64 L214 L215 L211 L206 L207 L208 L209 L253 L252 L251 L250 L249 L248 L246 L245 L244 L236 L237 L291 L290 L232 A9 L240 L239 L238 L243 L242 L188 L189 L199 L198 L197 L196 L35 L36 L37 L32 L38 L39 L40 L41 L98 L103 L102 L101 L100 L99 L143 L144 L145 L141 L140 | L230 A9 A10 L232 L233 A8 | L230 L231 A10 A9 | A8 L349 L348 L347 L159 L158 L163 L118 L117 A10 L114 L113 L112 L154 L153 L149 L148 L147 L336 L337 | L233 L232 A10 L290 L289 A8 | A8 L347 L348 L349 | L289 L290 A10 L291 L286 A8 | L147 L148 L149 A10 | L286 L291 A10 L237 L247 L246 L248 L253 L209 L210 L211 L215 L213 A8 L254 L255 L256 L300 L299 L298 | A8 L163 L158 L159 | L298 L299 L300 A8 | L153 L154 A10 | A10 L246 L247 L237 | A8 L121 L116 A10 L117 L118 | L256 L255 L254 A8 | A8 L62 A10 L116 L121 | L112 L113 L114 A10 | A10 L253 L248 | A8 L65 A10 L62 | L213 L215 A10 L214 L216 A8 | A8 L216 L214 A10 L65 | A10 L211 L210 L209
extrude "押し出し2" add sketch "スケッチ2" along normal blind 9 contours A6 | A7
fillet "フィレット1" radius 2 12 edges at (-26.2641, 0, -108.9378) (-20.9321, 0, -120.9157) (-19.5608, 0, -133.9548) (-54.9645, 0, -145.5638) (-62.7291, 0, -116.586) (-26.2641, 10, -108.9378) (-20.9321, 10, -120.9157) (-19.5608, 10, -133.9548) (-54.9645, 10, -145.5638) (-62.7291, 10, -116.586) (-122.0965, 10, -148.0226) (-122.0965, 0, -148.0226)
fillet "フィレット2" radius 10 4 edges at (-86.5065, 9.4476, -153.3736) (-86.5065, 0.5524, -153.3736) (-93.9502, 0.5524, -125.5935) (-93.9502, 9.4476, -125.5935)
